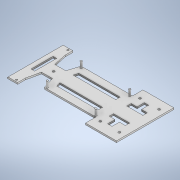
# Autodesk Inventor part: onderplaat final
Saved by Autodesk Inventor 2022 (Build 260153000, 153)
## iProperties
Created: 2022-10-31
Part Number: onderplaat final
Material: Generic
Document SubType Name: Modeling
Designer: devol
Density: 1 g/cm^3
Appearance: Default
Author: devol
Autodesk Inventor part; units mm, degrees
ref_plane "YZ Plane" through (0, 0, 0) normal (1, 0, 0) x (0, 1, 0)
ref_plane "XZ Plane" through (0, 0, 0) normal (0, 1, 0) x (-1, 0, 0)
ref_plane "XY Plane" through (0, 0, 0) normal (0, 0, 1) x (1, 0, 0)
sketch "Sketch1" plane through (0, 0, 0) normal (0, 1, 0) x (-1, 0, 0)
  line L0 (42, -64) -> (112, -64)
  line L1 (112, -64) -> (112, -14)
  line L2 (112, -14) -> (42, -14)
  line L3 (112, -39) -> (112, -30)
  line L4 (112, -39) -> (112, -48)
  line L5 (112, -30) -> (136, -30)
  line L6 (136, -30) -> (136, -48)
  line L7 (136, -48) -> (112, -48)
  line L8 (112, -30) -> (117, -30)
  line L9 (117, -30) -> (112, -14)
  line L10 (112, -48) -> (117, -48)
  line L11 (117, -48) -> (112, -64)
  line L12 (136, -30) -> (136, -1.5)
  line L13 (136, -1.5) -> (150, -1.5)
  line L14 (136, -48) -> (136, -76.5)
  line L15 (136, -76.5) -> (150, -76.5)
  line L16 (150, -76.5) -> (150, -1.5)
  line L17 (42, -14) -> (42, 0)
  line L18 (42, 0) -> (42, -78)
  line L19 (42, -78) -> (0, -78)
  line L20 (0, -78) -> (0, 0)
  line L21 (0, 0) -> (42, 0)
  line L22 (136, -30) -> (132, -30)
  line L23 (136, -30) -> (136, -12)
  line L24 (136, -12) -> (132, -30)
  line L25 (136, -48) -> (132, -48)
  line L26 (136, -48) -> (136, -66)
  line L27 (136, -66) -> (132, -48)
  dimension "d3" = 70
  dimension "d4" = 50
  dimension "d5" = 9
  dimension "d6" = 9
  dimension "d7" = 24
  dimension "d8" = 18
  dimension "d9" = 5
  dimension "d10" = 5
  dimension "d11" = 28.5
  dimension "d12" = 14
  dimension "d13" = 28.5
  dimension "d14" = 14
  dimension "d20" = 78
  dimension "d21" = 42
  dimension "d22" = 14
  dimension "d23" = 14
  dimension "d24" = 1.5
  dimension "d25" = 94
  dimension "d26" = 4
  dimension "d27" = 18
  dimension "d28" = 4
  dimension "d29" = 18
  constraints: 56 end point, 9 point on line, 7 perpendicular, 3 vertical, 1 horizontal, 1 midpoint
  measures "d3" distance of L0.start L0.end
  measures "d4" distance of L0.end L1.end
  measures "d5" distance of L3.start L3.end
  measures "d6" distance of L3.start L4.end
  measures "d7" distance of L3.end L5.end
  measures "d8" distance of L5.end L6.end
  measures "d9" distance of L3.end L8.end
  measures "d10" distance of L4.end L10.end
  measures "d11" distance of L5.end L12.end
  measures "d12" distance of L12.end L13.end
  measures "d13" distance of L6.end L14.end
  measures "d14" distance of L14.end L15.end
  measures "d20" distance of L17.end L18.end
  measures "d21" distance between parallel lines of L20 L17
  measures "d22" distance from line of L17.end L2
  measures "d23" distance from line of L18.end L0
  measures "d24" distance from line of L17.end L13
  measures "d25" distance between parallel lines of L18 L14
  measures "d26" distance of L5.end L22.end
  measures "d27" distance of L5.end L23.end
  measures "d28" distance of L6.end L25.end
  measures "d29" distance of L6.end L26.end
extrude "Extrusion1" add sketch "Sketch1" along normal blind 2.2
sketch "Sketch2" plane through (0, 2.2, 0) normal (0, 1, 0) x (1, 0, 0)
  circle A0 centre (-34, 12) radius 1.5
  circle A1 centre (-8, 12) radius 1.5
  line L0 (-42, 0) -> (0, 0) projected
  line L1 (0, 0) -> (0, 78) projected
  line L2 (-42, 14) -> (-42, 0) projected
  circle A2 centre (-34, 66) radius 1.5
  circle A3 centre (-8, 66) radius 1.5
  line L3 (-42, 78) -> (-42, 64) projected
  line L4 (0, 78) -> (-42, 78) projected
  circle A4 centre (-124.5, 39) radius 1.5
  line L5 (-132, 30) -> (-117, 30) projected
  circle A5 centre (-140, 4) radius 1.25
  line L6 (-136, 1.5) -> (-136, 12) projected
  line L7 (-150, 1.5) -> (-136, 1.5) projected
  circle A6 centre (-140, 74) radius 1.25
  line L8 (-136, 66) -> (-136, 76.5) projected
  line L9 (-136, 76.5) -> (-150, 76.5) projected
  line L10 (-142.75, 26.5) -> (-137.75, 26.5)
  line L11 (-137.75, 26.5) -> (-137.75, 56.5)
  line L12 (-137.75, 56.5) -> (-142.75, 56.5)
  line L13 (-142.75, 56.5) -> (-142.75, 26.5)
  line L14 (-150, 76.5) -> (-150, 1.5) projected
  dimension "d32" = 3
  dimension "d33" = 3
  dimension "d34" = 12
  dimension "d35" = 8
  dimension "d36" = 8
  dimension "d37" = 12
  dimension "d38" = 3
  dimension "d39" = 3
  dimension "d40" = 8
  dimension "d41" = 12
  dimension "d42" = 12
  dimension "d43" = 8
  dimension "d44" = 9
  dimension "d45" = 7.5
  dimension "d46" = 3
  dimension "d47" = 2.5
  dimension "d48" = 4
  dimension "d49" = 2.5
  dimension "d50" = 2.5
  dimension "d51" = 4
  dimension "d52" = 2.5
  dimension "d53" = 5
  dimension "d54" = 30
  dimension "d55" = 20
  dimension "d56" = 7.25
  constraints: 8 end point, 7 centre point, 2 parallel, 1 horizontal, 1 perpendicular
  measures "d32" diameter of A1
  measures "d33" diameter of A0
  measures "d34" distance from line of L0 A1.centre
  measures "d35" distance from line of L1 A1.centre
  measures "d36" distance from line of L2 A0.centre
  measures "d37" distance from line of L0 A0.centre
  measures "d38" diameter of A2
  measures "d39" diameter of A3
  measures "d40" distance from line of L3 A2.centre
  measures "d41" distance from line of L4 A2.centre
  measures "d42" distance from line of L4 A3.centre
  measures "d43" distance from line of L1 A3.centre
  measures "d44" distance from line of L5 A4.centre
  measures "d45" horizontal distance of L5.end A4.centre
  measures "d46" diameter of A4
  measures "d47" diameter of A5
  measures "d48" distance from line of L6 A5.centre
  measures "d49" distance from line of L7 A5.centre
  measures "d50" diameter of A6
  measures "d51" distance from line of L8 A6.centre
  measures "d52" distance from line of L9 A6.centre
  measures "d53" distance of L12.end L11.end
  measures "d54" distance of L11.end L10.end
  measures "d55" distance between parallel lines of L9 L12
  measures "d56" distance between parallel lines of L13 L14
extrude "Extrusion2" cut sketch "Sketch2" against normal blind 2.2
sketch "Sketch3" plane through (0, 2.2, 0) normal (0, 1, 0) x (1, 0, 0)
  line L0 (-42, 14) -> (-42, 0) projected
  line L1 (-42, 64) -> (-112, 64) projected
  line L2 (-42, 14) -> (-112, 14)
  line L3 (-112, 14) -> (-112, 64)
  line L4 (-112, 64) -> (-42, 64)
  line L5 (-42, 64) -> (-42, 14)
  circle A0 centre (-110, 16) radius 1.3
  circle A1 centre (-110, 62) radius 1.3
  circle A2 centre (-44, 16) radius 1.3
  circle A3 centre (-44, 62) radius 1.3
  point P0 (0, 0)
  dimension "d59" = 2
  dimension "d60" = 2
  dimension "d61" = 2.6
  dimension "d62" = 2
  dimension "d63" = 2
  dimension "d64" = 2.6
  dimension "d65" = 2.6
  dimension "d66" = 2.6
  dimension "d67" = 2
  dimension "d68" = 2
  dimension "d69" = 2
  dimension "d70" = 2
  constraints: 8 end point, 4 centre point, 2 parallel, 1 horizontal, 1 perpendicular
  measures "d59" distance from line of A0.centre L3
  measures "d60" distance from line of A0.centre L2
  measures "d61" diameter of A0
  measures "d62" distance from line of A1.centre L3
  measures "d63" distance from line of L1 A1.centre
  measures "d64" diameter of A1
  measures "d65" diameter of A2
  measures "d66" diameter of A3
  measures "d67" distance from line of A2.centre L2
  measures "d68" distance from line of L5 A2.centre
  measures "d69" distance from line of L1 A3.centre
  measures "d70" distance from line of L5 A3.centre
extrude "Extrusion3" add sketch "Sketch3" along normal blind 8 contours A0 | A1 | A2 | A3
sketch "Sketch4" plane through (0, 2.2, 0) normal (0, 1, 0) x (1, 0, 0)
  line L0 (-132, 30) -> (-117, 30) projected
  line L1 (-117, 30) -> (-112, 14) projected
  line L2 (-105.125, 24) -> (-107, 30)
  line L3 (-117, 48) -> (-132, 48) projected
  line L4 (-112, 64) -> (-117, 48) projected
  line L5 (-112, 64) -> (-102, 64)
  line L6 (-42, 64) -> (-112, 64) projected
  line L7 (-107, 48) -> (-105.125, 54)
  line L8 (-112, 14) -> (-42, 14) projected
  line L9 (-107, 30) -> (-49, 30)
  line L10 (-49, 30) -> (-49, 24)
  line L11 (-105.125, 24) -> (-49, 24)
  line L12 (-107, 48) -> (-49, 48)
  line L13 (-49, 48) -> (-49, 54)
  line L14 (-105.125, 54) -> (-49, 54)
  point P0 (0, 0)
  dimension "d79" = 10
  dimension "d88" = 10
  dimension "d93" = 10
  dimension "d111" = 58
  dimension "d112" = 6
  dimension "d113" = 10
  dimension "d114" = 6
  dimension "d115" = 72.646
  dimension "d116" = 58
  dimension "d117" = 56.125
  dimension "d118" = 18
  dimension "d119" = 6
  dimension "d120" = 6
  constraints: 18 end point, 3 horizontal, 1 point on line
  measures "d79" distance of L4.start L5.end
  measures "d88" distance of L0.end L2.end
  measures "d93" distance of L7.start L3.start
  measures "d111" distance of L2.end L9.end
  measures "d112" distance of L9.end L10.end
  measures "d113" distance between parallel lines of L8 L11
  measures "d114" distance between parallel lines of L9 L11
  measures "d115" angle of L9 L2
  measures "d116" distance of L7.start L12.end
  measures "d117" distance of L13.end L7.end
  measures "d118" distance between parallel lines of L9 L12
  measures "d119" distance of L13.end L12.end
  measures "d120" distance between parallel lines of L12 L14
extrude "Extrusion4" cut sketch "Sketch4" against normal blind 8
sketch "Sketch6" plane through (0, 2.2, 0) normal (0, 1, 0) x (1, 0, 0)
  line L0 (-34, 24) -> (-26, 24)
  line L1 (-26, 24) -> (-26, 14)
  line L2 (-26, 14) -> (-20, 14)
  line L3 (-34, 24) -> (-34, 30)
  line L4 (-34, 30) -> (-20, 30)
  line L5 (-20, 14) -> (-20, 24)
  line L6 (-20, 24) -> (-12, 24)
  line L7 (-12, 24) -> (-12, 30)
  line L8 (-12, 30) -> (-20, 30)
  line L9 (0, 0) -> (0, 78) projected
  line L10 (0, 39) -> (-41.084, 39)
  line L11 (-34, 54) -> (-26, 54)
  line L12 (-26, 54) -> (-26, 64)
  line L13 (-26, 64) -> (-20, 64)
  line L14 (-34, 54) -> (-34, 48)
  line L15 (-34, 48) -> (-20, 48)
  line L16 (-20, 64) -> (-20, 54)
  line L17 (-20, 54) -> (-12, 54)
  line L18 (-12, 54) -> (-12, 48)
  line L19 (-12, 48) -> (-20, 48)
  line L20 (-49, 30) -> (-49, 24) projected
  dimension "d97" = 8
  dimension "d98" = 10
  dimension "d99" = 6
  dimension "d100" = 16
  dimension "d101" = 6
  dimension "d102" = 10
  dimension "d103" = 8
  dimension "d104" = 6
  dimension "d105" = 9
  dimension "d121" = 15
  constraints: 38 end point, 9 symmetric about line, 6 perpendicular, 2 vertical, 1 horizontal, 1 midpoint
  measures "d97" distance of L0.start L0.end
  measures "d98" distance of L0.end L1.end
  measures "d99" distance of L1.end L2.end
  measures "d100" distance of L2.end L4.end
  measures "d101" distance of L0.start L3.end
  measures "d102" distance of L2.end L5.end
  measures "d103" distance of L5.end L6.end
  measures "d104" distance of L6.end L7.end
  measures "d105" distance between parallel lines of L10 L4
  measures "d121" distance between parallel lines of L3 L20
extrude "Extrusion5" cut sketch "Sketch6" against normal blind 8
chamfer "Chamfer1" distance 1 angle 45 1 edges at (-150, 2.2, -39)
body "Solid1"
